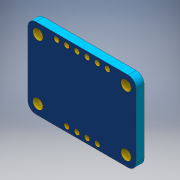
# Autodesk Inventor part: Adafruit 9-DOF Absolute Orientation IMU
Saved by Autodesk Inventor 2016 (Build 200138000, 138)
## iProperties
Created: 2016-05-24
Part Number: Adafruit 9-DOF Absolute Orientation IMU
Material: Generic
Document SubType Name: Modeling
Designer: Jacob
Density: 1 g/cm^3
Appearance: Default
Author: Jacob
Autodesk Inventor part; units mm, degrees
ref_plane "YZ Plane" through (0, 0, 0) normal (1, 0, 0) x (0, 1, 0)
ref_plane "XZ Plane" through (0, 0, 0) normal (0, 1, 0) x (-1, 0, 0)
ref_plane "XY Plane" through (0, 0, 0) normal (0, 0, 1) x (1, 0, 0)
sketch "Sketch1" plane through (0, 0, 0) normal (0, 1, 0) x (-1, 0, 0)
  line L0 (-13.5, 10) -> (13.5, 10)
  line L1 (13.5, 10) -> (13.5, -10)
  line L2 (13.5, -10) -> (-13.5, -10)
  line L3 (-13.5, -10) -> (-13.5, 10)
  line L4 (-13.5, 10) -> (13.5, -10) construction
  line L5 (13.5, 10) -> (-13.5, -10) construction
  point P0 (0, 0)
  dimension "d0" = 27
  dimension "d1" = 20
  constraints: 12 end point, 2 midpoint, 2 parallel, 1 horizontal, 1 perpendicular
  measures "d0" distance of L1.end L2.end
  measures "d1" distance of L0.end L1.end
extrude "Extrusion1" add sketch "Sketch1" along normal blind 4
sketch "Sketch2" plane through (0, 4, 0) normal (0, 1, 0) x (1, 0, 0)
  line L0 (-14.3189, -19.5529) -> (-14.3189, 19.8293) construction
  line L1 (-14.3189, 19.8293) -> (15.238, 19.8293) construction
  line L2 (15.238, 19.8293) -> (15.238, -19.5529) construction
  line L3 (15.238, -19.5529) -> (-14.3189, -19.5529) construction
  line L4 (-13.5, -10) -> (13.5, -10) projected
  line L5 (13.5, -10) -> (13.5, 10) projected
  line L6 (13.5, 10) -> (-13.5, 10) projected
  line L7 (-13.5, 10) -> (-13.5, -10) projected
  line L8 (-10.8374, -0.3883) -> (-2.9465, -0.3883)
  line L9 (-2.9465, -0.3883) -> (-2.9465, 3.5111)
  line L10 (-2.9465, 3.5111) -> (-10.8374, 3.5111)
  line L11 (-10.8374, 3.5111) -> (-10.8374, -0.3883)
  line L12 (-1.5955, -2.7525) -> (2.1811, -2.7525)
  line L13 (2.1811, -2.7525) -> (2.1811, 2.6207)
  line L14 (2.1811, 2.6207) -> (-1.5955, 2.6207)
  line L15 (-1.5955, 2.6207) -> (-1.5955, -2.7525)
  line L16 (-6.8919, 4.6778) -> (-5.0344, 4.6778)
  line L17 (-5.0344, 4.6778) -> (-5.0344, 5.9674)
  line L18 (-5.0344, 5.9674) -> (-6.8919, 5.9674)
  line L19 (-6.8919, 5.9674) -> (-6.8919, 4.6778)
  line L20 (-6.5081, -2.7525) -> (-4.451, -2.7525)
  line L21 (-4.451, -2.7525) -> (-4.451, -1.5551)
  line L22 (-4.451, -1.5551) -> (-6.5081, -1.5551)
  line L23 (-6.5081, -1.5551) -> (-6.5081, -2.7525)
  line L24 (-9.3022, -4.5641) -> (-7.9819, -4.5641)
  line L25 (-7.9819, -4.5641) -> (-7.9819, -1.77)
  line L26 (-7.9819, -1.77) -> (-9.3022, -1.77)
  line L27 (-9.3022, -1.77) -> (-9.3022, -4.5641)
  line L28 (-5.9632, -6.2221) -> (-4.8194, -6.2221)
  line L29 (-4.8194, -6.2221) -> (-4.8194, -3.6123)
  line L30 (-4.8194, -3.6123) -> (-5.9632, -3.6123)
  line L31 (-5.9632, -3.6123) -> (-5.9632, -6.2221)
  line L32 (-2.9465, -6.437) -> (-1.9946, -6.437)
  line L33 (-1.9946, -6.437) -> (-1.9946, -3.6123)
  line L34 (-1.9946, -3.6123) -> (-2.9465, -3.6123)
  line L35 (-2.9465, -3.6123) -> (-2.9465, -6.437)
  line L36 (-0.9814, -6.437) -> (0.2928, -6.437)
  line L37 (0.2928, -6.437) -> (0.2928, -3.8579)
  line L38 (0.2928, -3.8579) -> (-0.9814, -3.8579)
  line L39 (-0.9814, -3.8579) -> (-0.9814, -6.437)
  line L40 (1.0451, -6.437) -> (2.1811, -6.437)
  line L41 (2.1811, -6.437) -> (2.1811, -3.8579)
  line L42 (2.1811, -3.8579) -> (1.0451, -3.8579)
  line L43 (1.0451, -3.8579) -> (1.0451, -6.437)
  line L44 (4.4225, -6.0686) -> (5.4357, -6.0686)
  line L45 (5.4357, -6.0686) -> (5.4357, -3.8579)
  line L46 (5.4357, -3.8579) -> (4.4225, -3.8579)
  line L47 (4.4225, -3.8579) -> (4.4225, -6.0686)
  line L48 (6.8174, -5.3624) -> (8.7518, -5.3624)
  line L49 (8.7518, -5.3624) -> (8.7518, -4.4106)
  line L50 (8.7518, -4.4106) -> (6.8174, -4.4106)
  line L51 (6.8174, -4.4106) -> (6.8174, -5.3624)
  line L52 (7.4315, -2.7525) -> (9.1202, -2.7525)
  line L53 (9.1202, -2.7525) -> (9.1202, -1.77)
  line L54 (9.1202, -1.77) -> (7.4315, -1.77)
  line L55 (7.4315, -1.77) -> (7.4315, -2.7525)
  line L56 (7.4315, 0.1382) -> (9.5194, 0.1382)
  line L57 (9.5194, 0.1382) -> (9.5194, 1.2697)
  line L58 (9.5194, 1.2697) -> (7.4315, 1.2697)
  line L59 (7.4315, 1.2697) -> (7.4315, 0.1382)
  line L60 (7.1245, 2.9584) -> (8.9667, 2.9584)
  line L61 (8.9667, 2.9584) -> (8.9667, 3.8795)
  line L62 (8.9667, 3.8795) -> (7.1245, 3.8795)
  line L63 (7.1245, 3.8795) -> (7.1245, 2.9584)
  line L64 (4.1769, 0.1382) -> (5.4357, 0.1382)
  line L65 (5.4357, 0.1382) -> (5.4357, 1.0855)
  line L66 (5.4357, 1.0855) -> (4.1769, 1.0855)
  line L67 (4.1769, 1.0855) -> (4.1769, 0.1382)
  line L68 (3.6549, -2.1538) -> (5.4357, -2.1538)
  line L69 (5.4357, -2.1538) -> (5.4357, -0.6954)
  line L70 (5.4357, -0.6954) -> (3.6549, -0.6954)
  line L71 (3.6549, -0.6954) -> (3.6549, -2.1538)
  line L72 (3.6549, 2.4364) -> (5.2515, 2.4364)
  line L73 (5.2515, 2.4364) -> (5.2515, 3.5111)
  line L74 (5.2515, 3.5111) -> (3.6549, 3.5111)
  line L75 (3.6549, 3.5111) -> (3.6549, 2.4364)
  line L76 (3.1329, 5.0156) -> (5.098, 5.0156)
  line L77 (5.098, 5.0156) -> (5.098, 6.3052)
  line L78 (5.098, 6.3052) -> (3.1329, 6.3052)
  line L79 (3.1329, 6.3052) -> (3.1329, 5.0156)
  line L80 (-0.3443, 3.8795) -> (0.8608, 3.8795)
  line L81 (0.8608, 3.8795) -> (0.8608, 5.9674)
  line L82 (0.8608, 5.9674) -> (-0.3443, 5.9674)
  line L83 (-0.3443, 5.9674) -> (-0.3443, 3.8795)
  line L84 (-2.1482, 4.1559) -> (-0.9814, 4.1559)
  line L85 (-0.9814, 4.1559) -> (-0.9814, 6.1516)
  line L86 (-0.9814, 6.1516) -> (-2.1482, 6.1516)
  line L87 (-2.1482, 6.1516) -> (-2.1482, 4.1559)
  constraints: 160 end point, 40 parallel, 20 horizontal, 20 perpendicular, 18 point on line, 2 other
extrude "Extrusion2" cut sketch "Sketch2" against normal blind 1
sketch "Sketch3" plane through (0, 3, 0) normal (0, 1, 0) x (1, 0, 0)
  line L0 (11, -7.5) -> (-11, -7.5)
  line L1 (-11, -7.5) -> (-11, 7.5)
  line L2 (-11, 7.5) -> (11, 7.5)
  line L3 (11, 7.5) -> (11, -7.5)
  line L4 (11, -7.5) -> (-11, 7.5) construction
  line L5 (-11, -7.5) -> (11, 7.5) construction
  circle A0 centre (-11, -7.5) radius 1.25
  circle A1 centre (11, -7.5) radius 1.25
  circle A2 centre (11, 7.5) radius 1.25
  circle A3 centre (-11, 7.5) radius 1.25
  point P0 (0, 0)
  dimension "d31" = 22
  dimension "d32" = 15
  dimension "d33" = 2.5
  dimension "d34" = 2.5
  dimension "d35" = 2.5
  dimension "d36" = 2.5
  constraints: 12 end point, 4 centre point, 4 coincident, 2 midpoint, 2 parallel, 1 horizontal, 1 perpendicular
  measures "d31" distance of L1.end L2.end
  measures "d32" distance of L0.end L1.end
  measures "d33" diameter of A0
  measures "d34" diameter of A1
  measures "d35" diameter of A2
  measures "d36" diameter of A3
extrude "Extrusion3" cut sketch "Sketch3" against normal blind 5 contours A0 L1 L0 | L0 L1 A0 | A1 L3 L0 | L0 L3 A1 | A3 L2 L1 | L1 L2 A3 | A2 L2 L3 | L3 L2 A2
sketch "Sketch4" plane through (0, 3, 0) normal (0, 1, 0) x (1, 0, 0)
  circle A0 centre (-11, 7.5) radius 1.25 projected
  circle A1 centre (11, -7.5) radius 1.25 projected
  circle A2 centre (-11, -7.5) radius 1.25 projected
  circle A3 centre (11, 7.5) radius 1.25 projected
  line L0 (-2.9465, -0.3883) -> (-2.9465, 3.5111) projected
  line L1 (-10.8374, -0.3883) -> (-2.9465, -0.3883) projected
  line L2 (-10.8374, 3.5111) -> (-10.8374, -0.3883) projected
  line L3 (-2.9465, 3.5111) -> (-10.8374, 3.5111) projected
  line L4 (2.1811, -2.7525) -> (2.1811, 2.6207) projected
  line L5 (-1.5955, -2.7525) -> (2.1811, -2.7525) projected
  line L6 (-1.5955, 2.6207) -> (-1.5955, -2.7525) projected
  line L7 (2.1811, 2.6207) -> (-1.5955, 2.6207) projected
  line L8 (-7.9819, -4.5641) -> (-7.9819, -1.77) projected
  line L9 (-9.3022, -4.5641) -> (-7.9819, -4.5641) projected
  line L10 (-9.3022, -1.77) -> (-9.3022, -4.5641) projected
  line L11 (-7.9819, -1.77) -> (-9.3022, -1.77) projected
  line L12 (0.2928, -6.437) -> (0.2928, -3.8579) projected
  line L13 (-0.9814, -6.437) -> (0.2928, -6.437) projected
  line L14 (-0.9814, -3.8579) -> (-0.9814, -6.437) projected
  line L15 (0.2928, -3.8579) -> (-0.9814, -3.8579) projected
  line L16 (-4.8194, -6.2221) -> (-4.8194, -3.6123) projected
  line L17 (-5.9632, -6.2221) -> (-4.8194, -6.2221) projected
  line L18 (-5.9632, -3.6123) -> (-5.9632, -6.2221) projected
  line L19 (-4.8194, -3.6123) -> (-5.9632, -3.6123) projected
  line L20 (2.1811, -6.437) -> (2.1811, -3.8579) projected
  line L21 (1.0451, -6.437) -> (2.1811, -6.437) projected
  line L22 (1.0451, -3.8579) -> (1.0451, -6.437) projected
  line L23 (2.1811, -3.8579) -> (1.0451, -3.8579) projected
  line L24 (-1.9946, -6.437) -> (-1.9946, -3.6123) projected
  line L25 (-2.9465, -6.437) -> (-1.9946, -6.437) projected
  line L26 (-2.9465, -3.6123) -> (-2.9465, -6.437) projected
  line L27 (-1.9946, -3.6123) -> (-2.9465, -3.6123) projected
  line L28 (5.4357, -2.1538) -> (5.4357, -0.6954) projected
  line L29 (3.6549, -2.1538) -> (5.4357, -2.1538) projected
  line L30 (3.6549, -0.6954) -> (3.6549, -2.1538) projected
  line L31 (5.4357, -0.6954) -> (3.6549, -0.6954) projected
  line L32 (5.098, 5.0156) -> (5.098, 6.3052) projected
  line L33 (3.1329, 5.0156) -> (5.098, 5.0156) projected
  line L34 (3.1329, 6.3052) -> (3.1329, 5.0156) projected
  line L35 (5.098, 6.3052) -> (3.1329, 6.3052) projected
  line L36 (0.8608, 3.8795) -> (0.8608, 5.9674) projected
  line L37 (-0.3443, 3.8795) -> (0.8608, 3.8795) projected
  line L38 (-0.3443, 5.9674) -> (-0.3443, 3.8795) projected
  line L39 (0.8608, 5.9674) -> (-0.3443, 5.9674) projected
  line L40 (-4.451, -2.7525) -> (-4.451, -1.5551) projected
  line L41 (-6.5081, -2.7525) -> (-4.451, -2.7525) projected
  line L42 (-6.5081, -1.5551) -> (-6.5081, -2.7525) projected
  line L43 (-4.451, -1.5551) -> (-6.5081, -1.5551) projected
  line L44 (-5.0344, 4.6778) -> (-5.0344, 5.9674) projected
  line L45 (-6.8919, 4.6778) -> (-5.0344, 4.6778) projected
  line L46 (-6.8919, 5.9674) -> (-6.8919, 4.6778) projected
  line L47 (-5.0344, 5.9674) -> (-6.8919, 5.9674) projected
  line L48 (9.5194, 0.1382) -> (9.5194, 1.2697) projected
  line L49 (7.4315, 0.1382) -> (9.5194, 0.1382) projected
  line L50 (7.4315, 1.2697) -> (7.4315, 0.1382) projected
  line L51 (9.5194, 1.2697) -> (7.4315, 1.2697) projected
  line L52 (-0.9814, 4.1559) -> (-0.9814, 6.1516) projected
  line L53 (-2.1482, 4.1559) -> (-0.9814, 4.1559) projected
  line L54 (-2.1482, 6.1516) -> (-2.1482, 4.1559) projected
  line L55 (-0.9814, 6.1516) -> (-2.1482, 6.1516) projected
  line L56 (5.4357, -6.0686) -> (5.4357, -3.8579) projected
  line L57 (4.4225, -6.0686) -> (5.4357, -6.0686) projected
  line L58 (4.4225, -3.8579) -> (4.4225, -6.0686) projected
  line L59 (5.4357, -3.8579) -> (4.4225, -3.8579) projected
  line L60 (8.7518, -5.3624) -> (8.7518, -4.4106) projected
  line L61 (6.8174, -5.3624) -> (8.7518, -5.3624) projected
  line L62 (6.8174, -4.4106) -> (6.8174, -5.3624) projected
  line L63 (8.7518, -4.4106) -> (6.8174, -4.4106) projected
  line L64 (5.2515, 2.4364) -> (5.2515, 3.5111) projected
  line L65 (3.6549, 2.4364) -> (5.2515, 2.4364) projected
  line L66 (3.6549, 3.5111) -> (3.6549, 2.4364) projected
  line L67 (5.2515, 3.5111) -> (3.6549, 3.5111) projected
  line L68 (8.9667, 2.9584) -> (8.9667, 3.8795) projected
  line L69 (7.1245, 2.9584) -> (8.9667, 2.9584) projected
  line L70 (7.1245, 3.8795) -> (7.1245, 2.9584) projected
  line L71 (8.9667, 3.8795) -> (7.1245, 3.8795) projected
  line L72 (9.1202, -2.7525) -> (9.1202, -1.77) projected
  line L73 (7.4315, -2.7525) -> (9.1202, -2.7525) projected
  line L74 (7.4315, -1.77) -> (7.4315, -2.7525) projected
  line L75 (9.1202, -1.77) -> (7.4315, -1.77) projected
  line L76 (5.4357, 0.1382) -> (5.4357, 1.0855) projected
  line L77 (4.1769, 0.1382) -> (5.4357, 0.1382) projected
  line L78 (4.1769, 1.0855) -> (4.1769, 0.1382) projected
  line L79 (5.4357, 1.0855) -> (4.1769, 1.0855) projected
  line L80 (13.5, -10) -> (-13.5, -10) projected
  line L81 (13.5, 10) -> (13.5, -10) projected
  line L82 (-13.5, 10) -> (13.5, 10) projected
  line L83 (-13.5, -10) -> (-13.5, 10) projected
  line L84 (13.5, -10) -> (-13.5, -10) projected
  line L85 (0, -10) -> (0, -8.73)
  line L86 (0, -8.73) -> (-1.27, -8.73)
  line L87 (-1.27, -8.73) -> (-3.81, -8.73)
  line L88 (-3.81, -8.73) -> (-6.35, -8.73)
  line L89 (0, -8.73) -> (1.27, -8.73)
  line L90 (1.27, -8.73) -> (3.81, -8.73)
  line L91 (3.81, -8.73) -> (6.35, -8.73)
  line L92 (0, 10) -> (0, 8.73)
  line L93 (0, 8.73) -> (1.278, 8.73)
  line L94 (1.278, 8.73) -> (3.818, 8.73)
  line L95 (0, 8.73) -> (-1.27, 8.73)
  line L96 (-1.27, 8.73) -> (-3.81, 8.73)
  circle A4 centre (-6.35, -8.73) radius 0.635
  circle A5 centre (-3.81, -8.73) radius 0.635
  circle A6 centre (-1.27, -8.73) radius 0.635
  circle A7 centre (1.27, -8.73) radius 0.635
  circle A8 centre (3.81, -8.73) radius 0.635
  circle A9 centre (6.35, -8.73) radius 0.635
  circle A10 centre (-3.81, 8.73) radius 0.635
  circle A11 centre (-1.27, 8.73) radius 0.635
  circle A12 centre (1.278, 8.73) radius 0.635
  circle A13 centre (3.818, 8.73) radius 0.635
  point P0 (0, 0)
  dimension "d39" = 1.27
  dimension "d40" = 1.27
  dimension "d41" = 2.54
  dimension "d42" = 2.54
  dimension "d44" = 1.27
  dimension "d45" = 2.54
  dimension "d46" = 2.54
  dimension "d48" = 1.27
  dimension "d49" = 1.278
  dimension "d50" = 2.54
  dimension "d51" = 1.27
  dimension "d52" = 2.54
  dimension "d54" = 1.27
  dimension "d55" = 1.27
  dimension "d56" = 1.27
  dimension "d57" = 1.27
  dimension "d58" = 1.27
  dimension "d59" = 1.27
  dimension "d61" = 1.27
  dimension "d62" = 1.27
  dimension "d63" = 1.27
  dimension "d64" = 1.27
  constraints: 24 end point, 10 centre point, 6 point on line, 3 horizontal, 2 midpoint, 2 vertical, 1 perpendicular
  measures "d39" distance of L85.start L85.end
  measures "d40" distance of L85.end L86.end
  measures "d41" distance of L86.end L87.end
  measures "d42" distance of L87.end L88.end
  measures "d44" distance of L85.end L89.end
  measures "d45" distance of L89.end L90.end
  measures "d46" distance of L90.end L91.end
  measures "d48" distance of L92.start L92.end
  measures "d49" distance of L92.end L93.end
  measures "d50" distance of L93.end L94.end
  measures "d51" distance of L92.end L95.end
  measures "d52" distance of L95.end L96.end
  measures "d54" diameter of A4
  measures "d55" diameter of A5
  measures "d56" diameter of A6
  measures "d57" diameter of A7
  measures "d58" diameter of A8
  measures "d59" diameter of A9
  measures "d61" diameter of A10
  measures "d62" diameter of A11
  measures "d63" diameter of A12
  measures "d64" diameter of A13
extrude "Extrusion4" cut sketch "Sketch4" against normal blind 5 contours A13 | A12 L94 L93 | L93 L94 A12 | A10 | A11 L96 L95 | L95 L96 A11 | A4 | A5 L88 L87 | L87 L88 A5 | A6 L87 L86 | L86 L87 A6 | A9 | A8 L91 L90 | L90 L91 A8 | A7 L90 L89 | L89 L90 A7
fillet "Fillet1" radius 2 4 edges at (13.5, 1.5, 10) (13.5, 1.5, -10) (-13.5, 1.5, -10) (-13.5, 1.5, 10)
sketch "Sketch5" plane through (0, 0, 0) normal (0, -1, 0) x (1, 0, 0)
  arc A0 (-11.5, 10) -> (-13.5, 8) centre (-11.5, 8) ccw projected
  line L0 (-13.5, 8) -> (-13.5, -8) projected
  arc A1 (-13.5, -8) -> (-11.5, -10) centre (-11.5, -8) ccw projected
  line L1 (-11.5, -10) -> (11.5, -10) projected
  arc A2 (11.5, -10) -> (13.5, -8) centre (11.5, -8) ccw projected
  line L2 (13.5, -8) -> (13.5, 8) projected
  arc A3 (13.5, 8) -> (11.5, 10) centre (11.5, 8) ccw projected
  line L3 (11.5, 10) -> (-11.5, 10) projected
  circle A4 centre (1.278, -8.73) radius 0.635 projected
  circle A5 centre (-3.81, -8.73) radius 0.635 projected
  circle A6 centre (3.81, 8.73) radius 0.635 projected
  circle A7 centre (-1.27, 8.73) radius 0.635 projected
  circle A8 centre (-6.35, 8.73) radius 0.635 projected
  circle A9 centre (-3.81, 8.73) radius 0.635 projected
  circle A10 centre (1.27, 8.73) radius 0.635 projected
  circle A11 centre (6.35, 8.73) radius 0.635 projected
  circle A12 centre (-1.27, -8.73) radius 0.635 projected
  circle A13 centre (3.818, -8.73) radius 0.635 projected
  circle A14 centre (-11, -7.5) radius 1.25 projected
  circle A15 centre (11, 7.5) radius 1.25 projected
  circle A16 centre (-11, 7.5) radius 1.25 projected
  circle A17 centre (11, -7.5) radius 1.25 projected
  point P0 (0, 0)
extrude "Extrusion5" cut sketch "Sketch5" against normal blind 1
sketch "Sketch6" plane through (0, 4, 0) normal (0, 1, 0) x (1, 0, 0)
  line L0 (-2.9465, -0.3883) -> (-2.9465, 3.5111) projected
  line L1 (-2.9465, 3.5111) -> (-10.8374, 3.5111) projected
  line L2 (-10.8374, 3.5111) -> (-10.8374, -0.3883) projected
  line L3 (-10.8374, -0.3883) -> (-2.9465, -0.3883) projected
  line L4 (2.1811, -2.7525) -> (2.1811, 2.6207) projected
  line L5 (2.1811, 2.6207) -> (-1.5955, 2.6207) projected
  line L6 (-1.5955, 2.6207) -> (-1.5955, -2.7525) projected
  line L7 (-1.5955, -2.7525) -> (2.1811, -2.7525) projected
  point P0 (0, 0)
extrude "Extrusion6" add sketch "Sketch6" along normal blind 1
chamfer "Chamfer1" distance 1 angle 45 1 edges at (-2.9465, 5, -1.5614)
sketch "Sketch7" plane through (0, 3, 0) normal (0, 1, 0) x (1, 0, 0)
  circle A0 centre (-6.35, -8.73) radius 0.635 projected
  circle A1 centre (-3.81, -8.73) radius 0.635 projected
  circle A2 centre (-1.27, -8.73) radius 0.635 projected
  circle A3 centre (1.27, -8.73) radius 0.635 projected
  circle A4 centre (3.81, -8.73) radius 0.635 projected
  circle A5 centre (6.35, -8.73) radius 0.635 projected
  circle A6 centre (3.818, 8.73) radius 0.635 projected
  circle A7 centre (1.278, 8.73) radius 0.635 projected
  circle A8 centre (-1.27, 8.73) radius 0.635 projected
  circle A9 centre (-3.81, 8.73) radius 0.635 projected
  point P0 (0, 0)
  constraints: 10 coincident
body "Solid1"
